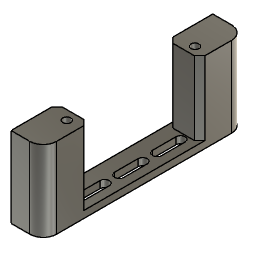
wanderer_mount v2 (Autodesk Fusion 360 design; units mm, degrees)
Autodesk Fusion 360 part; units mm, degrees
note: some values were not read from the file. Chosen so that the rebuilt part matches the saved one: a side.
sketch "Sketch1" plane through (0, 0, 0) normal (0, 0, 1) x (1, 0, 0)
  line L0 (0, 0) -> (12, 0)
  line L1 (12, 0) -> (12, 75.25)
  line L2 (12, 75.25) -> (0, 75.25)
  line L3 (0, 75.25) -> (0, 0)
  circle A0 centre (7.075, 13.705) radius 1.5
  circle A1 centre (7.075, 61.545) radius 1.5
  circle A2 centre (7.075, 13.705) radius 2.965 construction
  circle A3 centre (7.075, 61.545) radius 2.965 construction
  line L4 (7.075, 64.51) -> (7.075, 75.25) construction
  line L5 (7.075, 10.74) -> (7.075, 0) construction
  point P0 (7.075, 64.51)
  point P1 (7.075, 10.74)
  point P2 (10.04, 61.545)
  dimension "d3" = 75.25
  dimension "d4" = 12
  dimension "d8" = 5.93
  dimension "d9" = 3
  dimension "d10" = 10.74
  dimension "d11" = 1.96
  constraint horizontal L0
  constraint vertical L1
  constraint horizontal L2
  constraint vertical L3
  constraint coincident L0.start L3.end
  constraint concentric A0 A2
  constraint concentric A1 A3
  constraint equal A0 A1
  constraint equal A2 A3
  constraint vertical A0.centre A1.centre
  constraint coincident A3 P0
  constraint vertical A1.centre P0
  constraint coincident A2 P1
  constraint vertical A0.centre P1
  constraint coincident P0 L4.start
  constraint coincident L2 L4.end
  constraint perpendicular L2 L4
  constraint coincident P1 L5.start
  constraint coincident L0 L5.end
  constraint perpendicular L0 L5
  constraint equal L4 L5
  constraint coincident A3 P2
  constraint horizontal A1.centre P2
  measures "d3" distance of L0.end L1.end
  measures "d4" distance of L0.start L0.end
  measures "d8" diameter of A3
  measures "d9" diameter of A1
  measures "d10" distance of L2 P0
  measures "d11" distance of L1 P2
extrude "Extrude1" add sketch "Sketch1" along normal blind 30
sketch "Sketch2" plane through (0, 0, 30) normal (0, 0, 1) x (-1, 0, 0)
  circle A0 centre (-7.075, -13.705) radius 1.5
  circle A1 centre (-7.075, -61.545) radius 1.5
  line L0 (0, -75.25) -> (0, 0)
  line L1 (0, 0) -> (-12, 0)
  line L2 (-12, 0) -> (-12, -75.25)
  line L3 (-12, -75.25) -> (0, -75.25)
  line L4 (-7.075, -61.545) -> (-7.075, -13.705) construction
  line L5 (-5.375, -56.145) -> (-5.375, -47.3983)
  arc A2 (-5.375, -47.3983) -> (-8.775, -47.3983) centre (-7.075, -47.3983) ccw
  line L6 (-8.775, -47.3983) -> (-8.775, -56.145)
  arc A3 (-8.775, -56.145) -> (-5.375, -56.145) centre (-7.075, -56.145) ccw
  line L7 (-7.075, -56.145) -> (-7.075, -47.3983) construction
  line L8 (-5.375, -41.9983) -> (-5.375, -33.2517)
  arc A4 (-5.375, -33.2517) -> (-8.775, -33.2517) centre (-7.075, -33.2517) ccw
  line L9 (-8.775, -33.2517) -> (-8.775, -41.9983)
  arc A5 (-8.775, -41.9983) -> (-5.375, -41.9983) centre (-7.075, -41.9983) ccw
  line L10 (-7.075, -41.9983) -> (-7.075, -33.2517) construction
  line L11 (-5.375, -27.8517) -> (-5.375, -19.105)
  arc A6 (-5.375, -19.105) -> (-8.775, -19.105) centre (-7.075, -19.105) ccw
  line L12 (-8.775, -19.105) -> (-8.775, -27.8517)
  arc A7 (-8.775, -27.8517) -> (-5.375, -27.8517) centre (-7.075, -27.8517) ccw
  line L13 (-7.075, -27.8517) -> (-7.075, -19.105) construction
  line L14 (-2.767, -13.705) -> (-2.767, -19.105) construction
  line L15 (-2.767, -27.8517) -> (-2.767, -33.2517) construction
  line L16 (-2.767, -47.3983) -> (-2.767, -41.9983) construction
  line L17 (-2.767, -56.145) -> (-2.767, -61.545) construction
  point P0 (-7.075, -45.6983)
  point P1 (-7.075, -43.6983)
  dimension "d14" = 1.7
  dimension "d15" = 2
  constraint coincident A1.centre L4.start
  constraint coincident A0.centre L4.end
  constraint tangent L5 A2
  constraint tangent A2 L6
  constraint parallel L5 L6
  constraint tangent L6 A3
  constraint tangent L5 A3
  constraint coincident L4 A2.centre
  constraint parallel L4 L7
  constraint tangent L8 A4
  constraint tangent A4 L9
  constraint parallel L8 L9
  constraint tangent L9 A5
  constraint tangent L8 A5
  constraint coincident L4 A4.centre
  constraint parallel L4 L10
  constraint tangent L11 A6
  constraint tangent A6 L12
  constraint parallel L11 L12
  constraint tangent L12 A7
  constraint tangent L11 A7
  constraint coincident L4 A6.centre
  constraint parallel L4 L13
  constraint equal A2 A5
  constraint equal A5 A7
  constraint equal L5 L8
  constraint equal L8 L11
  constraint parallel L11 L15
  constraint parallel L5 L16
  constraint parallel L2 L17
  constraint horizontal A1.centre L17.end
  constraint horizontal A3.centre L17.start
  constraint vertical L16.start L17.start
  constraint horizontal A2.centre L16.start
  constraint horizontal A5.centre L16.end
  constraint vertical L15.end L16.end
  constraint horizontal A4.centre L15.end
  constraint horizontal A7.centre L15.start
  constraint horizontal A6.centre L14.end
  constraint vertical L14.end L15.start
  constraint vertical L14
  constraint horizontal A0.centre L14.start
  constraint equal L16 L17
  constraint equal L15 L16
  constraint equal L14 L15
  constraint midpoint A2 P0
  constraint midpoint A5 P1
  measures "d14" radius of A2
  measures "d15" distance of P0 P1
extrude "Extrude2" cut sketch "Sketch2" against normal up to surface (30 mm away) contours L5 A2 L6 A3 | L8 A4 L9 A5 | L11 A6 L12 A7
sketch "Sketch3" plane through (0, 0, 30) normal (0, 0, 1) x (-1, 0, 0)
  arc A0 (-8.775, -41.9983) -> (-5.375, -41.9983) centre (-7.075, -41.9983) ccw
  line L0 (-8.775, -41.9983) -> (-8.775, -33.2517)
  arc A1 (-5.375, -33.2517) -> (-8.775, -33.2517) centre (-7.075, -33.2517) ccw
  line L1 (-5.375, -33.2517) -> (-5.375, -41.9983)
  arc A2 (-8.775, -27.8517) -> (-5.375, -27.8517) centre (-7.075, -27.8517) ccw
  line L2 (-8.775, -27.8517) -> (-8.775, -19.105)
  arc A3 (-5.375, -19.105) -> (-8.775, -19.105) centre (-7.075, -19.105) ccw
  line L3 (-5.375, -19.105) -> (-5.375, -27.8517)
  arc A4 (-8.775, -56.145) -> (-5.375, -56.145) centre (-7.075, -56.145) ccw
  line L4 (-8.775, -56.145) -> (-8.775, -47.3983)
  arc A5 (-5.375, -47.3983) -> (-8.775, -47.3983) centre (-7.075, -47.3983) ccw
  line L5 (-5.375, -47.3983) -> (-5.375, -56.145)
  circle A6 centre (-7.075, -61.545) radius 1.5
  circle A7 centre (-7.075, -13.705) radius 1.5
  line L6 (0, -75.25) -> (0, 0)
  line L7 (0, 0) -> (-12, 0)
  line L8 (-12, 0) -> (-12, -75.25)
  line L9 (-12, -75.25) -> (0, -75.25)
  line L10 (-12, -17.1456) -> (0, -17.1456)
  line L11 (-12, -58.3399) -> (0, -58.3399)
  constraint coincident L8 L10.start
  constraint coincident L6 L10.end
  constraint perpendicular L6 L10
  constraint coincident L8 L11.start
  constraint coincident L6 L11.end
  constraint perpendicular L6 L11
extrude "Extrude3" cut sketch "Sketch3" against normal up to surface (27.4 mm away) contours L6 L8 L10 L11
chamfer "Chamfer1" distance 2 angle 45 4 edges at (12, 17.1456, 16.3) (0, 17.1456, 16.3) (12, 58.3399, 16.3) (0, 58.3399, 16.3)
fillet "Fillet1" radius 5 2 edges at (12, 0, 15) (12, 75.25, 15)
equation "bar_L = 75.25 mm"
equation "bar_W = 12 mm"
equation "d3 = bar_L"
equation "d4 = bar_W"
equation "M3_D = 3 mm"
equation "clearance = 0.2 mm"
equation "counterBore = 5.93 mm"
equation "d8 = counterBore"
equation "d9 = M3_D"
equation "d12 = bar_H"
equation "d14 = M3_D / 2 + clearance"
equation "d18 = bottom_t"
equation "bottom_t = 2.6 mm"
equation "bar_H = 30 mm"
